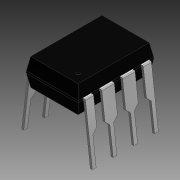
# Autodesk Inventor part: ATTiny85
Saved by Autodesk Inventor 2014 (Build 180170000, 170)
## iProperties
Created: 2013-11-20
Part Number: ATTiny85
Material: Generic
Document SubType Name: Modeling
Designer: Jesse
Density: 1 g/cm^3
Appearance: Default
Mass: 0.194382 g
Surface Area: 3.29361 cm^2
Volume: 0.194382 cm^3
Author: Jesse
Autodesk Inventor part; units mm, degrees
ref_plane "YZ Plane" through (0, 0, 0) normal (1, 0, 0) x (0, 1, 0)
ref_plane "XZ Plane" through (0, 0, 0) normal (0, 1, 0) x (-1, 0, 0)
ref_plane "XY Plane" through (0, 0, 0) normal (0, 0, 1) x (1, 0, 0)
sketch "Sketch1" plane through (0, 0, 0) normal (0, 1, 0) x (-1, 0, 0)
  line L0 (-3.175, -4.6355) -> (3.175, -4.6355)
  line L1 (3.175, -4.6355) -> (3.175, 4.6355)
  line L2 (3.175, 4.6355) -> (-3.175, 4.6355)
  line L3 (-3.175, 4.6355) -> (-3.175, -4.6355)
  line L4 (-3.175, -4.6355) -> (3.175, 4.6355) construction
  line L5 (3.175, -4.6355) -> (-3.175, 4.6355) construction
  point P0 (0, 0)
  dimension "d0" = 6.35
  dimension "d1" = 9.271
  constraints: 12 end point, 2 midpoint, 2 parallel, 1 horizontal, 1 perpendicular
  measures "d0" distance of L2.end L1.end
  measures "d1" distance of L0.end L1.end
extrude "Extrusion1" add sketch "Sketch1" along normal mid plane 3.302
ref_plane "Work Plane1" through (-3.175, 1.651, 4.0386) normal (0, 0, 1) x (1, 0, 0)
sketch "Sketch4" plane through (-3.175, 1.651, 4.0386) normal (0, 0, 1) x (1, 0, 0)
  line L0 (6.35, -3.302) -> (6.35, 0) projected
  line L1 (0, 0) -> (6.35, 0) projected
  line L2 (0, -3.302) -> (0, 0) projected
  line L3 (6.35, -3.302) -> (0, -3.302) projected
  line L4 (6.5405, -1.651) -> (6.5405, -1.524) construction
  line L5 (6.5405, -1.524) -> (6.35, -1.524)
  line L6 (6.35, -1.7721) -> (6.4273, -1.7721)
  line L7 (6.5405, -1.778) -> (6.1595, -1.524) construction
  line L8 (6.5405, -1.524) -> (6.1595, -1.778) construction
  line L9 (6.35, -1.651) -> (6.5405, -1.651) construction
  line L10 (6.5405, -1.651) -> (6.985, -5.3071) construction
  line L11 (6.5405, -1.651) -> (10.2235, -1.651) construction
  line L12 (6.35, -3.302) -> (6.35, 0) projected
  line L13 (6.985, -5.3071) -> (7.3835, -8.5849) construction
  line L14 (7.3835, -8.5849) -> (7.5096, -8.5696)
  line L15 (7.3835, -8.5849) -> (7.2574, -8.6003)
  line L16 (7.2574, -8.6003) -> (6.4273, -1.7721)
  line L17 (7.5096, -8.5696) -> (7.1111, -5.2918)
  line L18 (7.1111, -5.2918) -> (6.6666, -1.6357)
  arc A0 (6.6666, -1.6357) -> (6.5405, -1.524) centre (6.5405, -1.651) ccw
  line L19 (7.1111, -5.2918) -> (6.8589, -5.3224)
  point P0 (3.175, -1.651)
  point P1 (3.175, -3.302)
  dimension "d10" = 0.254
  dimension "d12" = 3.683
  dimension "d15" = 0.1905
  dimension "d16" = 3.302
  dimension "d17" = 0.127
  dimension "d18" = 0.127
  dimension "d19" = 3.302
  dimension "d20" = 3.683
  dimension "d52" = 3.81
  constraints: 30 end point, 7 midpoint, 5 perpendicular, 4 point on line, 3 collinear, 2 parallel, 2 point on circle, 1 centre point, 1 equal length, 1 horizontal, 1 tangent
  measures "d10" distance of L7.start L4.end
  measures "d12" distance of L4.start L10.end
  measures "d15" distance between parallel lines of L4 L0
  measures "d16" distance of L10.end L13.end
  measures "d17" distance of L13.end L14.end
  measures "d18" distance of L13.end L15.end
  measures "d19" distance of L14.end L17.end
  measures "d20" distance of L17.end L18.end
  measures "d52" horizontal distance of L10.end point (3.175, -3.302)
extrude "Extrusion3" add sketch "Sketch4" against normal blind 0.9906 contours L0 L5 A0 L18 L19 L16 L6
extrude "Extrusion4" add sketch "Sketch4" against normal blind 0.4572 contours L19 L17 L14 L15 L16
mirror "Mirror1" about plane through (0, 0, 0) normal (0, 0, 1) of "Extrusion4", "Extrusion3"
mirror "Mirror2" about plane through (0, 0, 0) normal (1, 0, 0) of "Extrusion3", "Extrusion4", "Mirror1"
ref_plane "Work Plane4" through (-3.175, 1.651, 1.27) normal (0, 0, 1) x (1, 0, 0)
ref_plane "Work Plane3" through (-3.175, 1.651, 3.81) normal (0, 0, 1) x (1, 0, 0)
sketch "Sketch6" plane through (-3.175, 1.651, 1.27) normal (0, 0, 1) x (1, 0, 0)
  line L0 (6.35, -3.2649) -> (6.35, 0)
  line L1 (0, 0) -> (6.35, 0)
  line L2 (0, -3.2649) -> (0, 0)
  line L3 (6.35, -3.2649) -> (0, -3.2649)
  line L4 (6.5405, -1.6325) -> (6.5405, -1.5099) construction
  line L5 (6.5405, -1.5099) -> (6.35, -1.5099)
  line L6 (6.35, -1.7536) -> (6.4273, -1.7536)
  line L7 (6.5405, -1.7639) -> (6.1696, -1.508) construction
  line L8 (6.5405, -1.5099) -> (6.1595, -1.755) construction
  line L9 (6.35, -1.6325) -> (6.5405, -1.6325) construction
  line L10 (6.5405, -1.6325) -> (6.985, -5.2885) construction
  line L11 (6.5405, -1.6325) -> (10.2235, -1.6325) construction
  line L12 (6.35, -3.2649) -> (6.35, 0)
  line L13 (6.985, -5.2885) -> (7.3835, -8.5664) construction
  line L14 (7.3835, -8.5664) -> (7.5096, -8.5511)
  line L15 (7.3835, -8.5664) -> (7.2574, -8.5817)
  line L16 (7.2574, -8.5817) -> (6.4273, -1.7536)
  line L17 (7.5096, -8.5511) -> (7.1111, -5.2732)
  line L18 (7.1111, -5.2732) -> (6.6666, -1.6171)
  arc A0 (6.6666, -1.6171) -> (6.5405, -1.5099) centre (6.5405, -1.6376) ccw
  line L19 (7.1111, -5.2732) -> (6.8589, -5.3039)
  line L20 (6.35, -3.302) -> (6.35, 0) projected
  line L21 (0, 0) -> (6.35, 0) projected
  line L22 (0, -3.302) -> (0, 0) projected
  line L23 (6.35, -3.302) -> (0, -3.302) projected
  line L24 (0, -3.302) -> (0, 0) projected
  point P0 (3.175, -1.651)
  point P1 (3.175, -1.651)
  point P2 (3.175, -3.302)
  dimension "d27" = 0.254
  dimension "d28" = 3.683
  dimension "d30" = 0.1905
  dimension "d31" = 3.302
  dimension "d32" = 0.127
  dimension "d33" = 0.127
  dimension "d34" = 3.302
  dimension "d35" = 3.683
  dimension "d53" = 3.81
  constraints: 40 end point, 8 perpendicular, 6 midpoint, 5 point on line, 3 collinear, 2 parallel, 2 point on circle, 1 centre point, 1 equal length, 1 horizontal, 1 tangent
  measures "d27" distance of L7.start L4.end
  measures "d28" distance of L4.start L10.end
  measures "d30" distance between parallel lines of L4 L0
  measures "d31" distance of L10.end L13.end
  measures "d32" distance of L13.end L14.end
  measures "d33" distance of L13.end L15.end
  measures "d34" distance of L14.end L17.end
  measures "d35" distance of L17.end L18.end
  measures "d53" horizontal distance of L10.end point (3.175, -3.302)
extrude "Extrusion5" add sketch "Sketch6" along normal mid plane 1.524 contours L0 L5 A0 L18 L19 L16 L6
extrude "Extrusion6" add sketch "Sketch6" along normal mid plane 0.4572 contours L19 L17 L14 L15 L16
mirror "Mirror3" about plane through (0, 0, 0) normal (0, 0, 1) of "Extrusion5", "Extrusion6"
mirror "Mirror4" about plane through (0, 0, 0) normal (1, 0, 0) of "Extrusion5", "Extrusion6", "Mirror3"
chamfer "Chamfer1" distance 1.524 angle 10 2 edges at (3.175, 1.651, 0) (3.175, -1.651, 0) measured on face at (3.175, 1.151, 0) measured on face at (3.175, -1.151, 0)
chamfer "Chamfer2" distance 1.524 angle 10 2 edges at (-3.175, 1.651, 0) (-3.175, -1.651, 0) measured on face at (-3.175, -1.151, 0) measured on face at (-3.175, 1.151, 0)
chamfer "Chamfer3" distance 1.524 angle 10 2 edges at (0, 1.651, 4.6355) (0, -1.651, 4.6355) measured on face at (0, 1.151, 4.6355) measured on face at (0, -1.151, 4.6355)
chamfer "Chamfer4" distance 1.524 angle 10 2 edges at (0, 1.651, -4.6355) (0, -1.651, -4.6355) measured on face at (0, -1.151, -4.6355) measured on face at (0, 1.151, -4.6355)
chamfer "Chamfer5" distance 0.5334 angle 45 12 edges at (3.81, -3.6375, 2.032) (3.81, -3.6375, 0.508) (3.81, -3.6561, 3.048) (3.81, -3.6375, -2.032) (3.81, -3.6375, -0.508) (3.81, -3.6561, -3.048) (-3.81, -3.6561, 3.048) (-3.81, -3.6375, 2.032) (-3.81, -3.6375, 0.508) (-3.81, -3.6375, -0.508) (-3.81, -3.6375, -2.032) (-3.81, -3.6561, -3.048)
sketch "Sketch7" plane through (0, 1.651, 0) normal (0, 1, 0) x (1, 0, 0)
  line L0 (2.9063, -4.3668) -> (-2.9063, -4.3668) projected
  line L1 (2.9063, 4.3668) -> (2.9063, -4.3668) projected
  circle A0 centre (1.8161, -3.2766) radius 0.2286
  line L2 (3.3655, -4.0386) -> (3.175, -4.0386) projected
  line L3 (3.3655, -4.0386) -> (3.3655, -3.048) projected
  line L4 (3.175, -3.048) -> (3.3655, -3.048) projected
  line L5 (3.175, -4.0386) -> (3.175, -3.048) projected
  point P0 (0, 0)
  dimension "d57" = 0.4572
  dimension "d58" = 0
  dimension "d59" = 1.0902
  dimension "d60" = 1.0902
  constraints: 1 centre point
  measures "d57" diameter of A0
  measures "d58" distance edge to line of A0 L4
  measures "d59" distance from line of L0 A0.centre
  measures "d60" distance from line of L1 A0.centre
extrude "Extrusion7" cut sketch "Sketch7" against normal blind 0.254 contours A0
equation "\"d53\" = d52"
equation "\"d60\" = d59"
body "Solid1"
